Autodesk Inventor part; units mm, degrees
(part 2 of 2)
  line L173 (99, -298) -> (91, -298)
  line L174 (152.4442, -54.0809) -> (152.4442, -2)
  line L175 (150.4442, -54.0809) -> (150.4442, -2)
  line L176 (149.6145, -54.4513) -> (135.1648, -41.4947)
  line L177 (148.2793, -55.9404) -> (133.8296, -42.9837)
  arc A124 (148.2793, -55.9404) -> (152.4442, -54.0809) centre (151.4442, -57.435) ccw
  arc A125 (150.4442, -54.0809) -> (149.6145, -54.4513) centre (151.4442, -57.435) ccw
  line L178 (99, -2) -> (91, -2)
  line L179 (89, -2) -> (68.2, -2)
  line L180 (152.4442, -263) -> (178.8, -263)
  line L181 (37.5558, -37) -> (11.2, -37)
  line L182 (11.2, -263) -> (37.5558, -263)
  line L183 (152.4442, -37) -> (178.8, -37)
  line L184 (152.4442, -36) -> (178.8, -36)
  line L185 (152.4442, -38) -> (178.8, -38)
  line L186 (37.5558, -36) -> (11.2, -36)
  line L187 (37.5558, -38) -> (11.2, -38)
  line L188 (152.4442, -262) -> (178.8, -262)
  line L189 (152.4442, -264) -> (178.8, -264)
  line L190 (11.2, -262) -> (37.5558, -262)
  line L191 (11.2, -264) -> (37.5558, -264)
  line L192 (23.1809, -231.5442) -> (11.2, -231.5442)
  arc A126 (24.1314, -228) -> (23.1809, -229.5442) centre (26.535, -230.5442) ccw
  arc A127 (23.1809, -231.5442) -> (27.7378, -227.2573) centre (26.535, -230.5442) ccw
  point P0 (0, 0)
  dimension "d490" = 2
  dimension "d496" = 2
  dimension "d505" = 2
  dimension "d513" = 2
  dimension "d562" = 2
  dimension "d590" = 35
  dimension "d591" = 35
  dimension "d592" = 35
  dimension "d593" = 35
  dimension "d594" = 1
  dimension "d595" = 1
  dimension "d596" = 1
  dimension "d597" = 1
  dimension "d598" = 1
  dimension "d599" = 1
  dimension "d600" = 1
  dimension "d601" = 1
  dimension "d605" = 2
  constraints: 324 end point, 178 point on circle, 86 centre point, 30 parallel, 9 perpendicular, 9 point on line, 5 horizontal, 1 midpoint
  measures "d490" distance between parallel lines of L21 L33
  measures "d496" distance between parallel lines of L5 L38
  measures "d505" distance between parallel lines of L13 L45
  measures "d513" distance between parallel lines of L3 L51
  measures "d562" distance between parallel lines of L22 L54
  measures "d590" distance between parallel lines of L180 L52
  measures "d591" distance between parallel lines of L182 L96
  measures "d592" distance between parallel lines of L130 L181
  measures "d593" distance between parallel lines of L183 L55
  measures "d594" distance between parallel lines of L183 L184
  measures "d595" distance between parallel lines of L183 L185
  measures "d596" distance between parallel lines of L181 L186
  measures "d597" distance between parallel lines of L181 L187
  measures "d598" distance between parallel lines of L180 L188
  measures "d599" distance between parallel lines of L180 L189
  measures "d600" distance between parallel lines of L182 L190
  measures "d601" distance between parallel lines of L182 L191
  measures "d605" distance between parallel lines of L192 L100
sketch "스케치30" plane through (0, 4, 0) normal (0, 1, 0) x (1, 0, 0)
  line L0 (229, -260) -> (229, -300) projected
  line L1 (229, -300) -> (230, -300) projected
  line L2 (230, -300) -> (230, -260) projected
  line L3 (230, -260) -> (229, -260) projected
  line L4 (229, 0) -> (229, -40) projected
  line L5 (229, -40) -> (230, -40) projected
  line L6 (230, -40) -> (230, 0) projected
  line L7 (230, 0) -> (229, 0) projected
  line L8 (-39, -40) -> (-39, 0) projected
  line L9 (-39, 0) -> (-40, 0) projected
  line L10 (-40, 0) -> (-40, -40) projected
  line L11 (-40, -40) -> (-39, -40) projected
  line L12 (-39, -300) -> (-39, -260) projected
  line L13 (-39, -260) -> (-40, -260) projected
  line L14 (-40, -260) -> (-40, -300) projected
  line L15 (-40, -300) -> (-39, -300) projected
  line L16 (230, -300) -> (230, -260) projected
  line L17 (230, -300) -> (190, -300)
  line L18 (190, -300) -> (190, -260)
  line L19 (190, -260) -> (230, -260)
  line L20 (230, -260) -> (230, -300)
  line L21 (230, 0) -> (229, 0) projected
  line L22 (230, 0) -> (190, 0)
  line L23 (190, 0) -> (190, -40)
  line L24 (190, -40) -> (230, -40)
  line L25 (230, -40) -> (230, 0)
  line L26 (-40, 0) -> (0, 0)
  line L27 (0, 0) -> (0, -40)
  line L28 (0, -40) -> (-40, -40)
  line L29 (-40, -40) -> (-40, 0)
  line L30 (-40, -300) -> (0, -300)
  line L31 (0, -300) -> (0, -260)
  line L32 (0, -260) -> (-40, -260)
  line L33 (-40, -260) -> (-40, -300)
  point P0 (0, 0)
  constraints: 32 end point, 8 parallel, 4 horizontal, 4 perpendicular
extrude "돌출29" cut sketch "스케치30" against normal blind 10
sketch "스케치31" plane through (0, 4, 0) normal (0, 1, 0) x (1, 0, 0)
  line L0 (17.1, -32) -> (17.1, -27) projected
  line L1 (17.1, -27) -> (27.1, -27) projected
  line L2 (27.1, -27) -> (27.1, -32) projected
  line L3 (27.1, -32) -> (17.1, -32) projected
  circle A0 centre (27.1, -23) radius 1.5 projected
  circle A1 centre (17.1, -23) radius 1.5 projected
  line L4 (12.1, -34) -> (32.1, -34) projected
  line L5 (32.1, -34) -> (32.1, -7) projected
  line L6 (32.1, -7) -> (12.1, -7) projected
  line L7 (12.1, -7) -> (12.1, -34) projected
  circle A2 centre (27.1, -13) radius 2.5 projected
  circle A3 centre (17.1, -13) radius 2.5 projected
  line L8 (162.9, -32) -> (162.9, -27) projected
  line L9 (162.9, -27) -> (172.9, -27) projected
  line L10 (172.9, -27) -> (172.9, -32) projected
  line L11 (172.9, -32) -> (162.9, -32) projected
  circle A4 centre (172.9, -23) radius 1.5 projected
  circle A5 centre (162.9, -23) radius 1.5 projected
  line L12 (157.9, -34) -> (177.9, -34) projected
  line L13 (177.9, -34) -> (177.9, -7) projected
  line L14 (177.9, -7) -> (157.9, -7) projected
  line L15 (157.9, -7) -> (157.9, -34) projected
  circle A6 centre (172.9, -13) radius 2.5 projected
  circle A7 centre (162.9, -13) radius 2.5 projected
  circle A8 centre (172.9, -287) radius 2.5 projected
  line L16 (172.9, -268) -> (172.9, -273) projected
  line L17 (172.9, -273) -> (162.9, -273) projected
  line L18 (162.9, -273) -> (162.9, -268) projected
  line L19 (162.9, -268) -> (172.9, -268) projected
  circle A9 centre (162.9, -277) radius 1.5 projected
  circle A10 centre (172.9, -277) radius 1.5 projected
  line L20 (177.9, -266) -> (157.9, -266) projected
  line L21 (157.9, -266) -> (157.9, -293) projected
  line L22 (157.9, -293) -> (177.9, -293) projected
  line L23 (177.9, -293) -> (177.9, -266) projected
  circle A11 centre (162.9, -287) radius 2.5 projected
  line L24 (27.1, -268) -> (27.1, -273) projected
  line L25 (27.1, -273) -> (17.1, -273) projected
  line L26 (17.1, -273) -> (17.1, -268) projected
  line L27 (17.1, -268) -> (27.1, -268) projected
  circle A12 centre (17.1, -277) radius 1.5 projected
  circle A13 centre (27.1, -277) radius 1.5 projected
  line L28 (32.1, -266) -> (12.1, -266) projected
  line L29 (12.1, -266) -> (12.1, -293) projected
  line L30 (12.1, -293) -> (32.1, -293) projected
  line L31 (32.1, -293) -> (32.1, -266) projected
  line L32 (27.1, -268) -> (27.1, -273) projected
  line L33 (27.1, -273) -> (17.1, -273) projected
  line L34 (17.1, -273) -> (17.1, -268) projected
  line L35 (17.1, -268) -> (27.1, -268) projected
  circle A14 centre (17.1, -277) radius 1.5 projected
  circle A15 centre (27.1, -277) radius 1.5 projected
  line L36 (32.1, -266) -> (12.1, -266) projected
  line L37 (12.1, -266) -> (12.1, -293) projected
  line L38 (12.1, -293) -> (32.1, -293) projected
  line L39 (32.1, -293) -> (32.1, -266) projected
  circle A16 centre (27.1, -287) radius 2.5 projected
  circle A17 centre (17.1, -287) radius 2.5 projected
  line L40 (12.1, -8) -> (32.1, -8)
  line L41 (32.1, -8) -> (32.1, -18)
  line L42 (32.1, -18) -> (12.1, -18)
  line L43 (12.1, -18) -> (12.1, -8)
  line L44 (157.9, -8) -> (177.9, -8)
  line L45 (177.9, -8) -> (177.9, -18)
  line L46 (177.9, -18) -> (157.9, -18)
  line L47 (157.9, -18) -> (157.9, -8)
  line L48 (157.9, -282) -> (177.9, -282)
  line L49 (177.9, -282) -> (177.9, -292)
  line L50 (177.9, -292) -> (157.9, -292)
  line L51 (157.9, -292) -> (157.9, -282)
  line L52 (32.1, -282) -> (12.1, -282)
  line L53 (12.1, -282) -> (12.1, -292)
  line L54 (12.1, -292) -> (32.1, -292)
  line L55 (32.1, -292) -> (32.1, -282)
  point P0 (0, 0)
  dimension "d571" = 20
  dimension "d572" = 10
  dimension "d573" = 5
  dimension "d574" = 5
  dimension "d575" = 20
  dimension "d576" = 10
  dimension "d577" = 5
  dimension "d578" = 5
  dimension "d579" = 20
  dimension "d580" = 10
  dimension "d581" = 5
  dimension "d582" = 5
  dimension "d583" = 20
  dimension "d584" = 10
  dimension "d585" = 5
  dimension "d586" = 5
  constraints: 32 end point, 8 parallel, 4 horizontal, 4 perpendicular
  measures "d571" distance of L41.end L42.end
  measures "d572" distance of L40.end L41.end
  measures "d573" distance from line of L40 A2.centre
  measures "d574" distance from line of L41 A2.centre
  measures "d575" distance of L45.end L46.end
  measures "d576" distance of L44.end L45.end
  measures "d577" distance from line of L47 A7.centre
  measures "d578" distance from line of L44 A7.centre
  measures "d579" distance of L49.end L50.end
  measures "d580" distance of L48.end L49.end
  measures "d581" distance from line of L48 A8.centre
  measures "d582" distance from line of L49 A8.centre
  measures "d583" distance of L54.end L53.end
  measures "d584" distance of L53.end L52.end
  measures "d585" distance from line of A17.centre L52
  measures "d586" distance from line of L53 A17.centre
extrude "돌출30" cut sketch "스케치31" against normal blind 4 contours A0 | A1 | L7 L40 L5 L42 | A2 | A3 | A4 | A5 | L15 L44 L13 L46 | A6 | A7 | A8 | A9 | A10 | L23 L50 L21 L48 | A11 | A12 | A13 | L31 L54 L29 L52 | A16 | A17
extrude "돌출31" cut sketch "스케치29" against normal blind 3.3 contours A79 L92 A76 L36 L95 L31 | L32 A65 L71 A59 L68 A58 L38 A53 L66 A50 L64 L75 L73 A61 L78 A63 L77 L53 | L33 L172 L166 A120 L169 L167 L83 A69 L82 A68 | L34 A77 L90 A73 L88 L168 L170 A122 L163 L171 | L97 L101 L102 L99 A81 L100 | L35 A75 L93 A80 L94 L190 L97 L192 A127 L98 L105 A82 L108 A86 L109 L89 A74 L91 A78 | L94 L182 L97 L190 | L37 A57 L69 A60 L70 A66 L54 A67 L81 A70 L84 L87 A71 L85 A56 | L39 A51 L111 A90 L112 A49 L67 A54 | L40 A55 L86 A72 L114 A89 L110 A52 | L56 L175 A125 L176 A45 L41 | A44 L177 A124 L174 L185 L57 L58 A47 L61 L65 A48 L113 A88 L149 L154 A115 L157 A43 L42 | L174 L183 L57 L185 | A42 L156 A114 L155 L148 L145 A111 L143 L144 L43 | L179 L140 A112 L146 L147 L151 A117 L152 A105 L44 | L45 A102 L128 A100 L123 L134 L131 A106 L137 A108 L135 L129 | L46 A104 L153 A116 L150 L160 A118 L158 A92 L48 A93 L126 A99 L127 A103 | L47 L133 L187 L136 A109 L138 A107 | L133 L181 L136 L187 | A91 L159 A119 L161 A87 L116 A98 L49 | A97 L118 A85 L107 A83 L120 A96 L50 | A95 L122 A84 L104 L132 L124 A101 L125 A94 L51 | L180 L76 L188 L74 | L188 L76 A64 L79 A62 L72 L74 | L59 L62 L63 L60 A46 | L139 L178 L142 A110 L141 A113 | A123 L164 A121 L165 L173 L162
